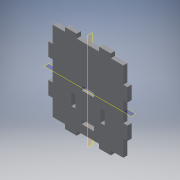
# Autodesk Inventor part: Part12
Saved by Autodesk Inventor 2018 (Build 220112000, 112)
## iProperties
Created: 2018-05-22
Part Number: Part12
Material: Generic
Document SubType Name: Modeling
Designer: Administrator
Density: 1 g/cm^3
Appearance: Default
Author: Administrator
Autodesk Inventor part; units mm, degrees
ref_plane "YZ Plane" through (0, 0, 0) normal (1, 0, 0) x (0, 1, 0)
ref_plane "XZ Plane" through (0, 0, 0) normal (0, 1, 0) x (-1, 0, 0)
ref_plane "XY Plane" through (0, 0, 0) normal (0, 0, 1) x (1, 0, 0)
sketch "Sketch1" plane through (0, 0, 0) normal (0, 0, 1) x (1, 0, 0)
  line L0 (-110.675, 126.35) -> (-171, 126.35)
  line L1 (-171, 126.35) -> (-171, 59.04)
  line L2 (-171, 59.04) -> (-110.675, 59.04)
  line L3 (-110.675, 59.04) -> (-110.675, 126.35)
  point P0 (0, 0)
  dimension "d0" = 60.325
  dimension "d1" = 67.31
  constraints: 8 end point, 2 parallel, 1 horizontal, 1 perpendicular
  measures "d0" distance between parallel lines of L1 L3
  measures "d1" distance between parallel lines of L2 L0
extrude "Extrusion1" add sketch "Sketch1" along normal blind 3.175
sketch "Sketch2" plane through (0, 0, 3.175) normal (0, 0, 1) x (1, 0, 0)
  line L0 (-171, 126.35) -> (-171, 59.04) projected
  line L1 (-171, 59.04) -> (-167.825, 59.04)
  line L2 (-167.825, 59.04) -> (-167.825, 74.915)
  line L3 (-167.825, 74.915) -> (-171, 74.915)
  line L4 (-171, 74.915) -> (-171, 59.04)
  line L5 (-171, 85.075) -> (-167.825, 85.075)
  line L6 (-167.825, 85.075) -> (-167.825, 100.315)
  line L7 (-167.825, 100.315) -> (-171, 100.315)
  line L8 (-171, 100.315) -> (-171, 85.075)
  line L9 (-110.675, 126.35) -> (-171, 126.35) projected
  line L10 (-171, 126.35) -> (-167.825, 126.35)
  line L11 (-167.825, 126.35) -> (-167.825, 110.475)
  line L12 (-167.825, 110.475) -> (-171, 110.475)
  line L13 (-171, 110.475) -> (-171, 126.35)
  point P0 (0, 0)
  dimension "d4" = 3.175
  dimension "d5" = 15.875
  dimension "d6" = 10.16
  dimension "d7" = 15.875
  dimension "d8" = 10.16
  constraints: 24 end point, 6 parallel, 3 horizontal, 3 perpendicular, 1 point on line
  measures "d4" distance between parallel lines of L0 L2
  measures "d5" distance between parallel lines of L3 L1
  measures "d6" distance between parallel lines of L3 L5
  measures "d7" distance between parallel lines of L9 L12
  measures "d8" distance between parallel lines of L12 L7
extrude "Extrusion3" cut sketch "Sketch2" against normal blind 3.175
ref_plane "Work Plane1" through (-140.8375, 59.04, 0) normal (1, 0, 0) x (0, 0, -1)
mirror "Mirror1" about plane through (-140.8375, 59.04, 0) normal (1, 0, 0) of "Extrusion3"
sketch "Sketch3" plane through (0, 0, 3.175) normal (0, 0, 1) x (1, 0, 0)
  line L0 (-123.375, 59.04) -> (-110.675, 59.04)
  line L1 (-110.675, 59.04) -> (-110.675, 62.215)
  line L2 (-110.675, 62.215) -> (-123.375, 62.215)
  line L3 (-123.375, 62.215) -> (-123.375, 59.04)
  line L4 (-167.825, 59.04) -> (-113.85, 59.04) projected
  line L5 (-110.675, 74.915) -> (-110.675, 85.075) projected
  line L6 (-140.8375, 59.04) -> (-132.265, 59.04)
  line L7 (-132.265, 59.04) -> (-132.265, 62.215)
  line L8 (-132.265, 62.215) -> (-140.8375, 62.215)
  line L9 (-140.8375, 62.215) -> (-140.8375, 59.04)
  point P0 (0, 0)
  dimension "d13" = 12.7
  dimension "d14" = 3.175
  dimension "d15" = 8.89
  constraints: 16 end point, 4 parallel, 2 collinear, 2 horizontal, 2 perpendicular, 1 midpoint
  measures "d13" distance between parallel lines of L3 L1
  measures "d14" distance between parallel lines of L0 L2
  measures "d15" distance between parallel lines of L3 L7
extrude "Extrusion4" cut sketch "Sketch3" against normal blind 3.175
mirror "Mirror2" about plane through (-140.8375, 59.04, 0) normal (1, 0, 0) of "Extrusion4"
ref_plane "Work Plane2" through (-158.3, 92.695, 0) normal (0, -1, 0) x (1, 0, 0)
mirror "Mirror3" about plane through (-158.3, 92.695, 0) normal (0, -1, 0) of "Extrusion4", "Mirror2"
sketch "Sketch4" plane through (0, 0, 3.175) normal (0, 0, 1) x (1, 0, 0)
  line L0 (-128.1375, 68.565) -> (-153.5375, 68.565)
  line L1 (-153.5375, 68.565) -> (-153.5375, 93.965)
  line L2 (-153.5375, 93.965) -> (-128.1375, 93.965)
  line L3 (-128.1375, 93.965) -> (-128.1375, 68.565)
  line L4 (-149.41, 62.215) -> (-132.265, 62.215) projected
  line L5 (-140.8375, 151.62) -> (-140.8375, -25.27) projected
  line L6 (-136.075, 93.965) -> (-145.6, 93.965)
  line L7 (-145.6, 93.965) -> (-145.6, 90.79)
  line L8 (-145.6, 90.79) -> (-136.075, 90.79)
  line L9 (-136.075, 90.79) -> (-136.075, 93.965)
  line L10 (-136.075, 68.565) -> (-145.6, 68.565)
  line L11 (-145.6, 68.565) -> (-145.6, 71.74)
  line L12 (-145.6, 71.74) -> (-136.075, 71.74)
  line L13 (-136.075, 71.74) -> (-136.075, 68.565)
  line L14 (-128.1375, 76.5025) -> (-131.3125, 76.5025)
  line L15 (-131.3125, 76.5025) -> (-131.3125, 86.0275)
  line L16 (-131.3125, 86.0275) -> (-128.1375, 86.0275)
  line L17 (-128.1375, 86.0275) -> (-128.1375, 76.5025)
  line L18 (-153.5375, 76.5025) -> (-150.3625, 76.5025)
  line L19 (-150.3625, 76.5025) -> (-150.3625, 86.0275)
  line L20 (-150.3625, 86.0275) -> (-153.5375, 86.0275)
  line L21 (-153.5375, 86.0275) -> (-153.5375, 76.5025)
  point P0 (0, 0)
  dimension "d18" = 6.35
  dimension "d19" = 12.7
  dimension "d20" = 25.4
  dimension "d21" = 25.4
  dimension "d22" = 7.9375
  dimension "d23" = 7.9375
  dimension "d24" = 3.175
  dimension "d25" = 3.175
  dimension "d26" = 7.9375
  dimension "d27" = 7.9375
  dimension "d28" = 3.175
  dimension "d29" = 3.175
  constraints: 40 end point, 10 parallel, 5 horizontal, 5 perpendicular, 4 point on line
  measures "d18" distance between parallel lines of L4 L0
  measures "d19" distance between parallel lines of L5 L1
  measures "d20" distance between parallel lines of L0 L2
  measures "d21" distance between parallel lines of L1 L3
  measures "d22" distance between parallel lines of L3 L9
  measures "d23" distance between parallel lines of L1 L7
  measures "d24" distance between parallel lines of L2 L8
  measures "d25" distance between parallel lines of L10 L12
  measures "d26" distance between parallel lines of L0 L14
  measures "d27" distance between parallel lines of L2 L16
  measures "d28" distance between parallel lines of L3 L15
  measures "d29" distance between parallel lines of L21 L19
extrude "Extrusion5" cut sketch "Sketch4" against normal blind 3.175 contours L0 L5 L12 L13 | L14 L15 L16 L3 | L0 L11 L12 L5 | L8 L7 L2 L5 | L5 L2 L9 L8 | L1 L20 L19 L18
body "Solid1"
